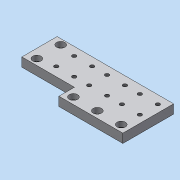
# Autodesk Inventor part: BC-10014
Saved by Autodesk Inventor 2016 (Build 200138000, 138)
## iProperties
Created: 2015-11-26
Part Number: BC-10014
Project: DIPOLO BC-3T- SIRIUS
Cost Center: 1504002005
Material: Alumínio 7075
Document SubType Name: Modeling
Designer: reinaldo.basilio
Density: 2.81 g/cm^3
Appearance: Satin - Brushed Heavy
Mass: 557.916 g
Surface Area: 428.174 cm^2
Volume: 198.547 cm^3
Description: Fixador dos blocos magnéticos.
RuleStatus: InUse
AfterMaterialChange0: file://_iMaterial
AfterAnyiPropertyChange0: file://_iMaterial
AfterDocNew0: file://_Naming_par
AfterDocNew1: file://_NameStart
AfterDocNew2: file://_NameStart1
AfterDocNew3: file://_Materiais
DocNumber: XXXXX-XXX-XXXX-00-001.ipt
Folder: .
Title: DIPOLO BC-3T- SIRIUS
Author: reinaldo.basilio
Subject: BC-10014
Autodesk Inventor part; units mm, degrees
ref_plane "YZ Plane" through (0, 0, 0) normal (1, 0, 0) x (0, 1, 0)
ref_plane "XZ Plane" through (0, 0, 0) normal (0, 1, 0) x (-1, 0, 0)
ref_plane "XY Plane" through (0, 0, 0) normal (0, 0, 1) x (1, 0, 0)
sketch "Sketch5" plane through (0, 0, 0) normal (0, 0, 1) x (1, 0, 0)
  line L0 (-42.5, 97.5) -> (42.5, 97.5)
  line L1 (42.5, 97.5) -> (42.5, -97.5)
  line L2 (42.5, -97.5) -> (-42.5, -97.5)
  line L3 (-42.5, -97.5) -> (-42.5, 97.5)
  point P0 (0, 0)
  point P1 (0, 97.5)
  point P2 (42.5, 0)
  point P3 (-42.5, 0)
  dimension "d8" = 195
  dimension "d9" = 85
  constraints: 8 end point, 3 midpoint, 2 horizontal alignment, 2 parallel, 1 horizontal, 1 perpendicular, 1 vertical alignment
  measures "d8" distance of L2.end L0.start
  measures "d9" distance of L0.start L0.end
extrude "Extrusion5" add sketch "Sketch5" along normal mid plane 15
sketch "Sketch6" plane through (0, 0, 7.5) normal (0, 0, 1) x (1, 0, 0)
  line L0 (42.5, -97.5) -> (16.5, -97.5)
  line L1 (16.5, -97.5) -> (16.5, -9.5)
  line L2 (16.5, -9.5) -> (42.5, -9.5)
  line L3 (42.5, -9.5) -> (42.5, -97.5)
  point P0 (0, 0)
  dimension "d12" = 88
  dimension "d13" = 26
  constraints: 8 end point, 2 parallel, 1 horizontal, 1 perpendicular
  measures "d12" distance of L0.end L1.end
  measures "d13" distance of L1.end L2.end
extrude "Extrusion6" cut sketch "Sketch6" against normal blind 15
sketch "Sketch7" plane through (0, 0, 7.5) normal (0, 0, 1) x (1, 0, 0)
  line L0 (42.5, 97.5) -> (-42.5, 97.5) projected
  line L1 (-42.5, 97.5) -> (-42.5, -97.5) projected
  line L2 (-42.5, -97.5) -> (16.5, -97.5) projected
  circle A0 centre (31.5, 83.75) radius 4.25
  circle A1 centre (31.5, 43.75) radius 4.25
  circle A2 centre (31.5, 3.75) radius 4.25
  circle A3 centre (-33.5, -82.5) radius 4.25
  circle A4 centre (6.5, -82.5) radius 4.25
  line L3 (16.5, -97.5) -> (16.5, -9.5) projected
  line L4 (42.5, -9.5) -> (42.5, 97.5) projected
  point P0 (0, 0)
  dimension "d17" = 74
  dimension "d18" = 8.5
  dimension "d19" = 40
  dimension "d20" = 40
  dimension "d21" = 13.75
  dimension "d22" = 40
  dimension "d23" = 15
  dimension "d66" = 10
  dimension "d68" = 11
  constraints: 5 centre point, 4 equal radius, 2 vertical alignment, 1 horizontal alignment
  measures "d17" distance from line of A0.centre L1
  measures "d18" diameter of A0
  measures "d19" distance of A0.centre A1.centre
  measures "d20" distance of A1.centre A2.centre
  measures "d21" distance from line of L0 A0.centre
  measures "d22" distance of A4.centre A3.centre
  measures "d23" distance from line of A4.centre L2
  measures "d66" distance from line of L3 A4.centre
  measures "d68" distance from line of L4 A0.centre
hole "Hole1" at (31.5, 83.75, 7.5) at (31.5, 43.75, 7.5) at (31.5, 3.75, 7.5) at (6.5, -82.5, 7.5) at (-33.5, -82.5, 7.5) direction (0, 0, -1) diameter 8.5 end through all counterbore diameter 14 counterbore depth 9 clearance for "Socket Head Cap Screw DIN EN ISO 4762" size "M8" standard "DIN"
sketch "Sketch8" plane through (0, 0, 7.5) normal (0, 0, 1) x (1, 0, 0)
  line L0 (42.5, 97.5) -> (-42.5, 97.5) projected
  line L1 (-42.5, 97.5) -> (-42.5, -97.5) projected
  line L2 (-42.5, -97.5) -> (16.5, -97.5) projected
  circle A0 centre (-28.5, 85) radius 4
  circle A1 centre (1.5, 85) radius 4
  circle A2 centre (-28.5, 55) radius 4
  circle A3 centre (1.5, 55) radius 4
  circle A4 centre (-28.5, 30) radius 4
  circle A5 centre (-28.5, 0) radius 4
  circle A6 centre (1.5, 30) radius 4
  circle A7 centre (1.5, 0) radius 4
  circle A8 centre (-28.5, -55) radius 4
  circle A9 centre (1.5, -55) radius 4
  line L3 (-57.3365, -67.5) -> (43.3911, -67.5)
  line L4 (-57.3365, -12.5) -> (43.3911, -12.5)
  line L5 (-57.3365, 42.5) -> (43.3911, 42.5)
  circle A10 centre (-28.5, -25) radius 4
  circle A11 centre (1.5, -25) radius 4
  point P0 (0, 0)
  dimension "d33" = 8
  dimension "d34" = 30
  dimension "d36" = 55
  dimension "d37" = 55
  dimension "d38" = 30
  dimension "d39" = 55
  dimension "d40" = 12.5
  dimension "d41" = 12.5
  dimension "d42" = 30
  dimension "d43" = 12.5
  dimension "d44" = 30
  dimension "d45" = 30
  dimension "d46" = 14
  constraints: 12 centre point, 12 vertical alignment, 11 equal radius, 6 end point, 6 horizontal alignment, 2 parallel, 1 horizontal
  measures "d33" diameter of A0
  measures "d34" distance of A2.centre A0.centre
  measures "d36" distance between parallel lines of L3 L4
  measures "d37" distance between parallel lines of L4 L5
  measures "d38" distance between parallel lines of L2 L3
  measures "d39" distance between parallel lines of L0 L5
  measures "d40" distance from line of L0 A0.centre
  measures "d41" distance from line of L5 A4.centre
  measures "d42" distance of A5.centre A4.centre
  measures "d43" distance from line of L3 A8.centre
  measures "d44" distance of A10.centre A8.centre
  measures "d45" distance of A1.centre A0.centre
  measures "d46" distance from line of A0.centre L1
hole "Hole2" at (-28.5, 85, 7.5) at (1.5, 85, 7.5) at (1.5, 55, 7.5) at (-28.5, 55, 7.5) at (-28.5, 30, 7.5) at (1.5, 30, 7.5) at (1.5, 0, 7.5) at (-28.5, 0, 7.5) at (-28.5, -25, 7.5) at (1.5, -25, 7.5) at (1.5, -55, 7.5) at (-28.5, -55, 7.5) direction (0, 0, -1) diameter 6.647 end through all thread size "M8x1.25" class "6H" standard "ISO Metric profile"
sketch "Sketch9" plane through (-42.5, -97.5, 7.5) normal (-1, 0, 0) x (0, 0, 1)
  line L0 (-15, 195) -> (0, 195)
  circle A0 centre (-7.5, 167.5) radius 3
  circle A1 centre (-7.5, 112.5) radius 3
  circle A2 centre (-7.5, 57.5) radius 3
  line L1 (0, 0) -> (-15, 0) projected
  point P0 (-7.5, 97.5)
  point P1 (-7.5, 97.5)
  dimension "d55" = 55
  dimension "d56" = 55
  dimension "d57" = 6
  dimension "d65" = 57.5
  constraints: 3 centre point, 3 vertical alignment, 2 end point, 2 equal radius
  measures "d55" distance of A1.centre A0.centre
  measures "d56" distance of A2.centre A1.centre
  measures "d57" diameter of A2
  measures "d65" distance from line of A2.centre L1
hole "Hole3" at (-42.5, -40, 0) at (-42.5, 15, 0) at (-42.5, 70, 0) direction (1, 0, 0) diameter 4.917 depth 15 tip angle 118 thread size "M6x1" class "6H" standard "ISO Metric profile"
equation "\"d20\" = d19"
body "Solid5"
